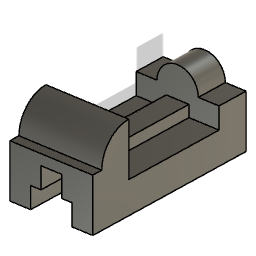
2) (Autodesk Fusion 360 design; units mm, degrees)
Autodesk Fusion 360 part; units mm, degrees
sketch "Sketch1" plane through (0, 0, 0) normal (0, 0, 1) x (1, 0, 0)
  line L0 (0, 0) -> (-170, 0)
  line L1 (-170, 0) -> (-170, -80)
  line L2 (-170, -80) -> (0, -80)
  line L3 (0, -80) -> (0, 0)
  dimension "d1" = 170
  dimension "d2" = 80
  constraint horizontal L0
  constraint vertical L1
  constraint horizontal L2
  constraint vertical L3
  constraint coincident L0.start L3.end
  measures "d1" distance of L0.start L0.end
  measures "d2" distance of L0.start L2.end
extrude "Extrude1" add sketch "Sketch1" along normal blind 30
sketch "Sketch2" plane through (0, 0, 30) normal (0, 0, 1) x (-1, 0, 0)
  line L0 (0, 80) -> (0, 0)
  line L1 (0, 0) -> (170, 0)
  line L2 (170, 0) -> (170, 80)
  line L3 (170, 80) -> (0, 80)
  line L4 (0, 80) -> (40, 80)
  line L5 (40, 80) -> (40, 0)
  line L6 (40, 0) -> (0, 0)
  line L7 (0, 0) -> (0, 80)
  dimension "d5" = 40
  constraint horizontal L4
  constraint vertical L5
  constraint horizontal L6
  constraint vertical L7
  constraint coincident L1 L5.end
  constraint coincident L0.start L3.end
  measures "d5" distance of L0.start L4.end
extrude "Extrude2" add sketch "Sketch2" along normal blind 50 contours L0 L1 L3 L4 L5 L6 L7
sketch "Sketch3" plane through (0, 0, 80) normal (0, 0, 1) x (-1, 0, 0)
  line L0 (0, 0) -> (40, 0)
  line L1 (40, 0) -> (40, 80)
  line L2 (40, 80) -> (0, 80)
  line L3 (0, 80) -> (0, 0)
  line L4 (0, 80) -> (10, 80)
  line L5 (10, 80) -> (10, 0)
  line L6 (10, 0) -> (0, 0)
  line L7 (0, 0) -> (0, 80)
  constraint horizontal L4
  constraint vertical L5
  constraint horizontal L6
  constraint vertical L7
  constraint coincident L0 L5.end
  constraint coincident L2.end L3.start
extrude "Extrude3" cut sketch "Sketch3" along normal blind 0 and the other way blind 30 contours L0 L2 L3 L4 L5 L6 L7
fillet "Fillet1" radius 30 1 edges at (-10, -40, 80)
sketch "Sketch4" plane through (0, 0, 30) normal (0, 0, 1) x (-1, 0, 0)
  line L0 (40, 80) -> (40, 0)
  line L1 (40, 0) -> (170, 0)
  line L2 (170, 0) -> (170, 80)
  line L3 (170, 80) -> (40, 80)
  line L4 (170, 80) -> (140, 80)
  line L5 (140, 80) -> (140, 0)
  line L6 (140, 0) -> (170, 0)
  line L7 (170, 0) -> (170, 80)
  constraint horizontal L4
  constraint vertical L5
  constraint horizontal L6
  constraint vertical L7
  constraint coincident L1 L5.end
  constraint coincident L2.end L3.start
extrude "Extrude4" add sketch "Sketch4" along normal blind 20 contours L1 L2 L3 L4 L5 L6 L7
sketch "Sketch5" plane through (-170, 0, 0) normal (-1, 0, 0) x (0, -1, 0)
  line L0 (0, 0) -> (80, 0)
  line L1 (80, 0) -> (80, 50)
  line L2 (80, 50) -> (0, 50)
  line L3 (0, 50) -> (0, 0)
  circle A0 centre (40, 50) radius 20
  dimension "d16" = 40
  constraint midpoint L2 A0.centre
  measures "d16" diameter of A0
extrude "Extrude5" add sketch "Sketch5" along normal blind 0 and the other way blind 30 contours L2 A0 picked at (45.5083, 53.7555)
sketch "Sketch6" plane through (0, 0, 30) normal (0, 0, 1) x (-1, 0, 0)
  line L0 (140, 0) -> (140, 80)
  line L1 (140, 80) -> (40, 80)
  line L2 (40, 80) -> (40, 0)
  line L3 (40, 0) -> (140, 0)
  line L4 (140, 50) -> (40, 50)
  line L5 (40, 50) -> (40, 30)
  line L6 (40, 30) -> (140, 30)
  line L7 (140, 30) -> (140, 50)
  constraint horizontal L4
  constraint vertical L5
  constraint horizontal L6
  constraint vertical L7
  constraint coincident L2 L5.end
  constraint coincident L0 L4.start
extrude "Extrude6" add sketch "Sketch6" along normal blind 10 contours L0 L2 L4 L5 L6 L7
sketch "Sketch7" plane through (0, 0, 0) normal (1, 0, 0) x (0, 1, 0)
  line L0 (0, 50) -> (-80, 50)
  line L1 (-80, 50) -> (-80, 0)
  line L2 (-80, 0) -> (0, 0)
  line L3 (0, 0) -> (0, 50)
  line L4 (-60, 0) -> (-20, 0)
  line L5 (-20, 0) -> (-20, 20)
  line L6 (-20, 20) -> (-60, 20)
  line L7 (-60, 20) -> (-60, 0)
  line L8 (-50, 20) -> (-30, 20)
  line L9 (-30, 20) -> (-30, 40)
  line L10 (-30, 40) -> (-50, 40)
  line L11 (-50, 40) -> (-50, 20)
  constraint horizontal L4
  constraint vertical L5
  constraint horizontal L6
  constraint vertical L7
  constraint coincident L2 L4.start
  constraint horizontal L8
  constraint vertical L9
  constraint horizontal L10
  constraint vertical L11
  constraint coincident L6 L8.start
extrude "Extrude7" cut sketch "Sketch7" along normal blind 0 and the other way blind 170 contours L2 L4 L5 L6 L7 L8 | L6 L8 L9 L10 L11
sketch "Sketch8" plane through (0, 0, 30) normal (0, 0, 1) x (-1, 0, 0)
  line L0 (140, 30) -> (40, 30)
  line L1 (40, 30) -> (40, 0)
  line L2 (40, 0) -> (140, 0)
  line L3 (140, 0) -> (140, 30)
  line L4 (40, 30) -> (140, 30)
  line L5 (140, 30) -> (140, 29)
  line L6 (140, 29) -> (40, 29)
  line L7 (40, 29) -> (40, 30)
  line L8 (40, 50) -> (140, 50)
  line L9 (140, 50) -> (140, 51)
  line L10 (140, 51) -> (40, 51)
  line L11 (40, 51) -> (40, 50)
  dimension "d27" = 1
  dimension "d28" = 100
  dimension "d29" = 1
  constraint horizontal L4
  constraint vertical L5
  constraint horizontal L6
  constraint vertical L7
  constraint coincident L0.end L1.start
  constraint horizontal L8
  constraint vertical L9
  constraint horizontal L10
  constraint vertical L11
  measures "d27" distance of L0.end L6.end
  measures "d28" distance of L8.start L8.end
  measures "d29" distance of L8.start L10.end
extrude "Extrude8" add sketch "Sketch8" along normal blind 10 contours L0 L1 L3 L4 L5 L6 L7 | L8 L9 L10 L11
sketch "Sketch9" plane through (0, 0, 40) normal (0, 0, 1) x (-1, 0, 0)
  line L0 (40, 29) -> (140, 29)
  line L1 (140, 29) -> (140, 30)
  line L2 (140, 30) -> (40, 30)
  line L3 (40, 30) -> (40, 29)
  line L4 (40, 51) -> (140, 51)
  line L5 (140, 51) -> (140, 29)
  line L6 (140, 29) -> (40, 29)
  line L7 (40, 29) -> (40, 51)
  constraint horizontal L4
  constraint vertical L5
  constraint horizontal L6
  constraint vertical L7
  constraint coincident L0.end L1.start
extrude "Extrude9" add sketch "Sketch9" along normal blind 1
